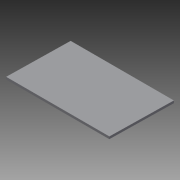
# Autodesk Inventor part: extDisplay
Saved by Autodesk Inventor 2017 (Build 210142000, 142)
## iProperties
Created: 2018-10-12
Part Number: extDisplay
Material: PC/ABS Plastic
Document SubType Name: Modeling
Designer: ari
Density: 0.357273 g/cm^3
Appearance: Smooth - White
Author: ari
Autodesk Inventor part; units mm, degrees
ref_plane "YZ Plane" through (0, 0, 0) normal (1, 0, 0) x (0, 1, 0)
ref_plane "XZ Plane" through (0, 0, 0) normal (0, 1, 0) x (-1, 0, 0)
ref_plane "XY Plane" through (0, 0, 0) normal (0, 0, 1) x (1, 0, 0)
sketch "Sketch1" plane through (0, 0, 0) normal (1, 0, 0) x (0, 1, 0)
  line L0 (0, 0) -> (235.1642, -4.1048)
  line L1 (235.1642, -4.1048) -> (235.0158, -12.6035)
  line L2 (235.0158, -12.6035) -> (-0.1483, -8.4987)
  line L3 (-0.1483, -8.4987) -> (0, 0)
  line L4 (-47.2109, 0) -> (282.2267, 0) construction
  dimension "d0" = 1
  dimension "d1" = 8.5
  dimension "d2" = 235.2
  constraints: 8 end point, 2 parallel, 1 perpendicular
  measures "d0" angle of L0 L4
  measures "d1" distance of L0.end L1.end
  measures "d2" distance of L1.end L2.end
extrude "Extrusion1" add sketch "Sketch1" along normal mid plane 376.2
body "Solid1"
